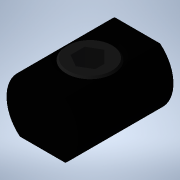
# Autodesk Inventor part: SCHUNK-9949504 limit stop for MMS-P
Saved by Autodesk Inventor 2021 (Build 250183000, 183)
## iProperties
Created: 2025-07-30
Part Number: SCHUNK-9949504 limit stop for MMS-P
Material: Generic
Catalog Web Link: www.cadenas.de
Description: Limit stop for MMS-P-ANS
Vendor: SCHUNK
Document SubType Name: Modeling
Designer: psAdmin
Manufacturer: SCHUNK
Mass: 0.0476436 g
Surface Area: 0.850002 cm^2
Volume: 0.0476436 cm^3
Density: 1 g/cm^3
Appearance: PSOLRGB-35-35-35
Category: PARTsolutions
Company: SCHUNK
Title: SCHUNK-9949504 limit stop for MMS-P
Author: Cadenas PARTsolutions
Comments: ANS
PSOL_IDENT_0: {$CADENAS_DATA/23d-libs/schunk/greifsysteme/zubehoer/sensorik/sensoren/magnetschalter/ans_mms_p.prj}
PSOL_IDENT_1: ,224 {VTYP=3D},{NB=SCHUNK-9949504 limit stop for MMS-P},{LINA=SCHUNK-9949504 limit stop for MMS-P},{
PSOL_IDENT_2: NN=Limit stop for MMS-P},{DATE=19.12.2024 14:49:43},{GEOMDATE=14.12.2022 07:37:41},{VERSION=},{LINEI
PSOL_IDENT_3: D=10},{WBVAR=},{WBNUMERIC=}  {NB=SCHUNK-9949504 Anschlag fuer MMS-P},{LINA=SCHUNK-9949504 Anschlag f
PSOL_IDENT_4: uer MMS-P},{KT=DUMMY},{IDNR=9949504},{TYP=MMS-P},{CNSCTN=84799070},{INFOXX=https://schunk.com/us/en/
PSOL_IDENT_5: p/000000000009949504}
NB: SCHUNK-9949504 limit stop for MMS-P
NN: Limit stop for MMS-P
NT: ANS
NBSYN: SCHUNK-$IDNR. limit stop for $TYP.
LINA: SCHUNK-9949504 limit stop for MMS-P
CATALOG: SCHUNK
IDNR: 9949504
TYP: MMS-P
CNSCTN: 84799070
SUPPLIER: SCHUNK
ARTICLENO: SCHUNK-9949504 limit stop for MMS-P
BOMINFO: SCHUNK-9949504 limit stop for MMS-P
CREATOR: CADENAS GmbH
Autodesk Inventor part; units mm, degrees
sketch "Sketch_1" plane through (0, 0, 0) normal (0, 0, 1) x (1, 0, 0)
  arc A0 (-1.1977, 2.95) -> (-1.1977, 0) centre (0, 1.475) ccw
  line L0 (-1.1977, 0) -> (1.1977, 0)
  arc A1 (1.1977, 0) -> (1.1977, 2.95) centre (0, 1.475) ccw
  line L1 (1.1977, 2.95) -> (-1.1977, 2.95)
  constraints: 4 end point, 4 point on circle, 2 centre point
extrude "Extrusion1" add sketch "Sketch_1" along normal mid plane 5
sketch "Sketch_2" plane through (0, 0, 0) normal (0, 0, 1) x (1, 0, 0)
  line L0 (0, 0) -> (0, 2.95)
  line L1 (1.15, 2.95) -> (1.25, 2.85)
  line L2 (1.25, 2.85) -> (1.25, 2.75)
  line L3 (1.25, 2.75) -> (1.45, 2.95)
  line L4 (1.45, 2.95) -> (1.15, 2.95)
  constraints: 10 end point
revolve "Revolution1" cut sketch "Sketch_2" angle 360 about axis through (0, 0, 0) along (0, -1, 0)
sketch "Sketch_3" plane through (0, 2.95, 0) normal (0, 1, 0) x (1, 0, 0)
  line L0 (-0.65, -0.3753) -> (0, -0.7506)
  line L1 (0, -0.7506) -> (0.65, -0.3753)
  line L2 (0.65, -0.3753) -> (0.65, 0.3753)
  line L3 (0.65, 0.3753) -> (0, 0.7506)
  line L4 (0, 0.7506) -> (-0.65, 0.3753)
  line L5 (-0.65, 0.3753) -> (-0.65, -0.3753)
  constraints: 12 end point
extrude "Extrusion2" cut sketch "Sketch_3" against normal blind 1.3
sketch "Sketch_5" plane through (0, 2.95, 0) normal (0, 1, 0) x (1, 0, 0)
  circle A0 centre (0, 0) radius 1.3
  constraints: 1 centre point
extrude "Extrusion3" cut sketch "Sketch_5" against normal blind 0.01
ref_plane "an_XY" through (0, 1.475, 2.5) normal (0, 0, 1) x (1, 0, 0)
ref_plane "an_YZ" through (0, 1.475, 2.5) normal (1, 0, 0) x (0, 1, 0)
ref_plane "an_ZX" through (0, 1.475, 2.5) normal (0, 1, 0) x (0, 0, 1)
ref_plane "ans_mms_p_XY" through (0, 1.475, 0) normal (0, 0, 1) x (1, 0, 0)
ref_plane "ans_mms_p_YZ" through (0, 1.475, 0) normal (1, 0, 0) x (0, 1, 0)
ref_plane "ans_mms_p_ZX" through (0, 1.475, 0) normal (0, 1, 0) x (0, 0, 1)
body "Solid1"
